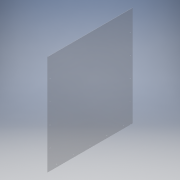
# Autodesk Inventor part: Short Wall
Saved by Autodesk Inventor 2017 (Build 210142000, 142)
## iProperties
Created: 2017-01-16
Part Number: Short Wall
Material: Polycarbonate, Clear
Document SubType Name: Modeling
Designer: Ben
Density: 1.2 g/cm^3
Appearance: Polycarbonate - Clear
Mass: 263.627 g
Surface Area: 2791.53 cm^2
Volume: 219.689 cm^3
Author: Ben
Autodesk Inventor part; units mm, degrees
ref_plane "YZ Plane" through (0, 0, 0) normal (1, 0, 0) x (0, 1, 0)
ref_plane "XZ Plane" through (0, 0, 0) normal (0, 1, 0) x (-1, 0, 0)
ref_plane "XY Plane" through (0, 0, 0) normal (0, 0, 1) x (1, 0, 0)
sketch "Sketch1" plane through (0, 0, 0) normal (1, 0, 0) x (0, 1, 0)
  line L0 (0, 0) -> (381, 0)
  line L1 (381, 0) -> (381, -323.85)
  line L2 (381, -323.85) -> (0, -323.85)
  line L3 (0, -323.85) -> (0, 0)
  line L4 (0, -314.325) -> (381, -314.325) construction
  line L5 (381, -161.925) -> (0, -161.925) construction
  line L6 (190.5, -323.85) -> (190.5, 0) construction
  line L7 (9.525, -323.85) -> (9.525, 0) construction
  circle A0 centre (9.525, -161.925) radius 1.5875
  circle A1 centre (9.525, -98.425) radius 1.5875
  circle A2 centre (9.525, -34.925) radius 1.5875
  circle A3 centre (9.525, -225.425) radius 1.5875
  circle A4 centre (9.525, -161.925) radius 1.5875
  circle A5 centre (9.525, -98.425) radius 1.5875
  circle A6 centre (9.525, -288.925) radius 1.5875
  circle A7 centre (9.525, -225.425) radius 1.5875
  circle A8 centre (9.525, -161.925) radius 1.5875
  circle A9 centre (190.5, -314.325) radius 1.5875
  circle A10 centre (273.05, -314.325) radius 1.5875
  circle A11 centre (355.6, -314.325) radius 1.5875
  circle A12 centre (107.95, -314.325) radius 1.5875
  circle A13 centre (25.4, -314.325) radius 1.5875
  line L8 (0, -9.525) -> (381, -9.525) construction
  circle A14 centre (190.5, -9.525) radius 1.5875
  circle A15 centre (273.05, -9.525) radius 1.5875
  circle A16 centre (355.6, -9.525) radius 1.5875
  circle A17 centre (107.95, -9.525) radius 1.5875
  circle A18 centre (25.4, -9.525) radius 1.5875
  dimension "d0" = 323.85
  dimension "d1" = 381
  dimension "d12" = 9.525
  dimension "d13" = 9.525
  dimension "d16" = 63.5
  dimension "d19" = 63.5
  dimension "d22" = 3.175
  dimension "d25" = 82.55
  dimension "d32" = 82.55
  constraints: 19 centre point, 18 end point, 7 midpoint, 7 symmetric about line, 5 point on line, 3 horizontal, 3 perpendicular, 2 parallel, 2 vertical, 1 equal radius, 29 other
  measures "d0" distance of L2.end L0.start
  measures "d1" distance of L0.start L0.end
  measures "d12" distance between parallel lines of L2 L4
  measures "d13" distance between parallel lines of L3 L7
  measures "d16" distance of A0.centre A1.centre
  measures "d19" distance of A0.centre A3.centre
  measures "d22" diameter of A0
  measures "d25" distance of A9.centre A10.centre
  measures "d32" distance of A9.centre A12.centre
extrude "Extrusion1" add sketch "Sketch1" along normal blind 1.5875
equation "\"d13\" = d12"
body "Solid1"
